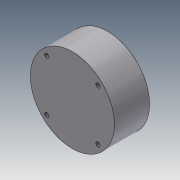
# Autodesk Inventor part: J008109
Saved by Autodesk Inventor 2018.3 (Build 223284000, 284)
## iProperties
Created: 2018-10-11
Material: ALUMINUM, 6061-T651
Vendor: HHMI: JRC - ID&F
Document SubType Name: Modeling
Designer: arnoldj
Density: 2.7 g/cm^3
Appearance: Metal-AL-6061 (Machined)
Part Number: J008109
Description: VP AIR CYLINFER MOUNT
Project: COMMON
RuleStatus: InUse
AfterDocSave0: file://Part Number Cleaner
LAB/DEPT: FLY FACILITY (SHARED RESOURCE)
REQUESTING SCIENTIST: LAVERTY, TODD
SURFACE ROUGHNESS: 64 Ra
DESIGN DEPARTMENT: HHMI: JRC - ID&F
SPECIAL FINISH: NONE
ALTERED ITEM PART NUMBER: N/A
ALTERED ITEM VENDOR: N/A
ALTERED ITEM DESCRIPTION: N/A
Author: arnoldj
Revision Number: -.1
Autodesk Inventor part; units mm, degrees
ref_plane "YZ Plane" through (0, 0, 0) normal (1, 0, 0) x (0, 1, 0)
ref_plane "XZ Plane" through (0, 0, 0) normal (0, 1, 0) x (-1, 0, 0)
ref_plane "XY Plane" through (0, 0, 0) normal (0, 0, 1) x (1, 0, 0)
sketch "Sketch1" plane through (0, 0, 0) normal (0, 0, 1) x (1, 0, 0)
  line L0 (0, 55.4736) -> (0, -55.4736) projected
  line L1 (-55.4736, 0) -> (55.4736, 0) projected
  circle A0 centre (0, 0) radius 39.624
  circle A1 centre (0, 0) radius 10.3188
  dimension "d0" = 20.6375
  dimension "d1" = 79.248
  constraints: 2 centre point, 2 coincident
  measures "d0" diameter of A1
  measures "d1" diameter of A0
extrude "Extrusion1" add sketch "Sketch1" along normal blind 26.924
sketch "Sketch2" plane through (0, 0, 0) normal (0, 0, -1) x (-1, 0, 0)
  line L0 (0, -55.4736) -> (0, 55.4736) projected
  line L1 (-55.4736, 0) -> (55.4736, 0) projected
  line L2 (-24.1554, -24.1554) -> (24.1554, -24.1554) construction
  line L3 (24.1554, -24.1554) -> (24.1554, 24.1554) construction
  line L4 (24.1554, 24.1554) -> (-24.1554, 24.1554) construction
  line L5 (-24.1554, 24.1554) -> (-24.1554, -24.1554) construction
  line L6 (-24.1554, -24.1554) -> (24.1554, 24.1554) construction
  line L7 (24.1554, -24.1554) -> (-24.1554, 24.1554) construction
  point P0 (0, 0)
  dimension "d22" = 48.3108
  constraints: 12 end point, 2 midpoint, 2 parallel, 2 perpendicular, 1 coincident, 1 horizontal
  measures "d22" distance of L3.end L4.end
hole "Hole1" at (-24.1554, -24.1554, 0) direction (0, 0, 1) diameter 4.1402 depth 14.1986 tip angle 118
sketch "Sketch3" plane through (0, 0, 26.924) normal (0, 0, 1) x (1, 0, 0)
  circle A0 centre (-24.1554, -24.1554) radius 2.0701 projected
  point P0 (0, 0)
  constraints: 1 coincident
hole "Hole2" at (-24.1554, -24.1554, 26.924) direction (0, 0, -1) diameter 4.1402 depth 14.1986 tip angle 118
pattern_circular "Circular Pattern1" count 4 over 360 about axis through (0, 0, -10) along (0, 0, 1) of "Hole1", "Hole2"
body "Solid1"
